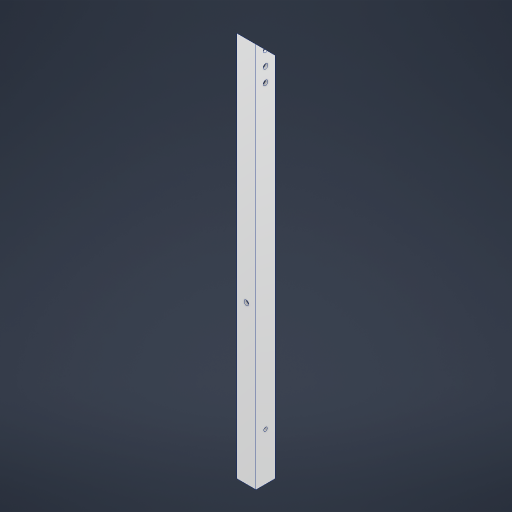
# Autodesk Inventor part: STRU_002_BilletPole_20.56in_Angled
Saved by Autodesk Inventor 2024.2 (Build 282272000, 272)
## iProperties
Created: 2024-07-23
Part Number: STRU_002_BilletPole_20.56in_Angled
Material: Aluminum 6061
Document SubType Name: Modeling
Designer: bryan
Density: 2.7 g/cm^3
Appearance: Aluminum - Flat
Mass: 386.313 g
Surface Area: 912.226 cm^2
Volume: 143.079 cm^3
Author: bryan
Autodesk Inventor part; units mm, degrees
ref_plane "YZ Plane" through (0, 0, 0) normal (1, 0, 0) x (0, 1, 0)
ref_plane "XZ Plane" through (0, 0, 0) normal (0, 1, 0) x (-1, 0, 0)
ref_plane "XY Plane" through (0, 0, 0) normal (0, 0, 1) x (1, 0, 0)
sketch "Sketch1" plane through (0, 0, 0) normal (0, 1, 0) x (-1, 0, 0)
  line L0 (-12.7, -12.7) -> (12.7, -12.7)
  line L1 (12.7, -12.7) -> (12.7, 12.7)
  line L2 (12.7, 12.7) -> (-12.7, 12.7)
  line L3 (-12.7, 12.7) -> (-12.7, -12.7)
  line L4 (-12.7, -12.7) -> (12.7, 12.7) construction
  line L5 (12.7, -12.7) -> (-12.7, 12.7) construction
  line L6 (9.525, 9.525) -> (9.525, -9.525)
  line L7 (9.525, -9.525) -> (-9.525, -9.525)
  line L8 (-9.525, -9.525) -> (-9.525, 9.525)
  line L9 (-9.525, 9.525) -> (9.525, 9.525)
  point P0 (0, 0)
  dimension "d0" = 25.4
  dimension "d1" = 25.4
  dimension "d2" = 3.175
  constraints: 20 end point, 4 parallel, 2 midpoint, 2 perpendicular, 1 horizontal, 3 other
  measures "d0" distance of L2.end L1.end
  measures "d1" distance of L1.end L0.end
  measures "d2" distance between parallel lines of L1 L6
extrude "Extrusion1" add sketch "Sketch1" along normal blind 514.35
sketch "Sketch2" plane through (12.7, 0, 12.7) normal (1, 0, 0) x (0, 0, -1)
  line L0 (25.4, 514.35) -> (0, 514.35) projected
  line L1 (0, 514.35) -> (25.4, 488.95)
  line L2 (25.4, 0) -> (25.4, 514.35) projected
  circle A0 centre (12.7, 482.6) radius 3.2512
  line L3 (0, 514.35) -> (25.4, 514.35) projected
  circle A1 centre (12.7, 463.55) radius 3.2512
  circle A2 centre (12.7, 501.65) radius 3.2512
  point P0 (12.7, 0)
  point P1 (12.7, 514.35)
  point P2 (12.7, 514.35)
  point P3 (14.9989, 499.3511)
  point P4 (10.4011, 503.9489)
  dimension "d5" = 25.4
  dimension "d6" = 6.5024
  dimension "d7" = 31.75
  dimension "d8" = 19.05
  constraints: 3 centre point, 3 midpoint, 2 end point, 2 equal radius, 2 vertical alignment, 1 point on line
  measures "d5" distance of L0.start L1.end
  measures "d6" diameter of A0
  measures "d7" distance of A0.centre point (12.7, 514.35)
  measures "d8" distance of A1.centre A0.centre
extrude "Extrusion2" cut sketch "Sketch2" against normal blind 522.224
sketch "Sketch5" plane through (12.7, 0, -12.7) normal (0, 0, -1) x (-1, 0, 0)
  circle A0 centre (12.7, 209.55) radius 3.2512
  line L0 (0, 0) -> (25.4, 0) projected
  line L1 (25.4, 514.35) -> (0, 514.35) projected
  point P0 (12.7, 0)
  point P1 (12.7, 0)
  point P2 (12.7, 514.35)
  dimension "d11" = 6.5024
  dimension "d15" = 304.8
  constraints: 2 midpoint, 1 centre point, 1 vertical alignment
  measures "d11" diameter of A0
  measures "d15" distance of A0.centre point (12.7, 514.35)
extrude "Extrusion3" cut sketch "Sketch5" against normal blind 25.4
sketch "Sketch6" plane through (-12.7, 0, -12.7) normal (-1, 0, 0) x (0, 0, 1)
  line L0 (12.7, 0) -> (12.7, 63.5)
  circle A0 centre (12.7, 63.5) radius 2.4892
  dimension "d16" = 63.5
  dimension "d17" = 4.9784
  constraints: 2 end point, 1 centre point, 1 coincident, 1 vertical
  measures "d16" distance of L0.start L0.end
  measures "d17" diameter of A0
extrude "Extrusion4" cut sketch "Sketch6" against normal blind 25.4
body "Solid1"
